linkage (Autodesk Fusion 360 design; units mm, degrees)
Autodesk Fusion 360 part; units mm, degrees
note: some values were not read from the file. Set by a fixed rule: which sketch regions a step uses.
sketch "Sketch1" plane through (0, 0, 0) normal (0, 0, 1) x (1, 0, 0)
  line L0 (15, -5) -> (-15, -5)
  line L1 (-15, -5) -> (-15, 5)
  line L2 (-15, 5) -> (15, 5)
  line L3 (15, 5) -> (15, -5)
  line L4 (15, -5) -> (-15, 5) construction
  line L5 (-15, -5) -> (15, 5) construction
  line L6 (15, 5) -> (15, 6)
  line L7 (-15, 5) -> (-15, 6)
  line L8 (-15, 6) -> (15, 6)
  circle A0 centre (15, 0) radius 5
  circle A1 centre (-15, 0) radius 5
  circle A2 centre (17.598076, -1.5) radius 0.75
  arc A3 (11.752405, -1.875) -> (18.247595, -1.875) centre (15, 0) ccw
  arc A4 (13.051443, -1.125) -> (11.752405, -1.875) centre (12.401924, -1.5) ccw
  arc A5 (13.051443, -1.125) -> (16.948557, -1.125) centre (15, 0) ccw
  arc A6 (18.247595, -1.875) -> (16.948557, -1.125) centre (17.598076, -1.5) ccw
  arc A7 (12.401924, -1.5) -> (17.598076, -1.5) centre (15, 0) ccw construction
  circle A8 centre (-15, 0) radius 1
  circle A9 centre (-13.341688, 2.5) radius 0.75
  circle A10 centre (15, 0) radius 0.85
  line L9 (10, 0) -> (10, 5)
  line L10 (10, 0) -> (10, -5)
  line L11 (-10, 0) -> (-10, 5)
  line L12 (-10, 0) -> (-10, -5)
  circle A11 centre (-13.341688, 2.5) radius 1.5
  circle A12 centre (17.598076, -1.5) radius 1.5
  spline S0 degree 5 poles (-13.906239, 3.889705) (-13.820569, 3.930394) (-13.594142, 4.00436) (-13.089374, 4.092943) (-12.082571, 4.167095) (-10.28252, 4.16815) (-7.990298, 4.046011) (-5.364162, 3.702697) (-2.588377, 3.078057) (0.216352, 2.217267) (2.95153, 1.211009) (5.549959, 0.187001) (7.964451, -0.719306) (10.166297, -1.382464) (12.141061, -1.714787) (13.885488, -1.67539) (15.098724, -1.33535) (15.908025, -0.90749) (16.403158, -0.545975) (16.639624, -0.34615) knots 0 0 0 0 0 0 0.06666667 0.13333333 0.2 0.26666667 0.33333333 0.4 0.46666667 0.53333333 0.6 0.66666667 0.73333333 0.8 0.86666667 0.93333333 1 1 1 1 1 1
  line L13 (-11.458957, 4.328773) -> (-4.541043, 3.671227)
  spline S1 degree 5 poles (-13.025243, 1.033759) (-12.77026, 1.082867) (-12.235105, 1.173979) (-11.356811, 1.289333) (-10.033525, 1.400235) (-8.132174, 1.457296) (-6.01483, 1.406336) (-3.754068, 1.195619) (-1.485479, 0.739596) (0.736265, 0.061952) (2.894168, -0.762718) (5.003407, -1.624735) (7.092733, -2.409171) (9.191281, -3.021107) (11.316096, -3.407147) (13.476739, -3.540705) (15.236985, -3.439146) (16.575337, -3.246285) (17.475584, -3.06623) (17.927711, -2.963332) knots 0 0 0 0 0 0 0.06666667 0.13333333 0.2 0.26666667 0.33333333 0.4 0.46666667 0.53333333 0.6 0.66666667 0.73333333 0.8 0.86666667 0.93333333 1 1 1 1 1 1
  line L14 (-8.520512, 1.622849) -> (-1.602599, 0.965303)
  point P0 (-8, 4)
  point P1 (9.308019, -1.092546)
  point P2 (-5.061556, 1.294076)
  point P3 (6.721235, -2.240412)
  dimension "d1" = 30
  dimension "d2" = 10
  dimension "d5" = 1
  dimension "d6" = 1
  dimension "d7" = 1.5
  dimension "d8" = 3
  dimension "d9" = 1.5
  dimension "d10" = 2
  dimension "d11" = 1.5
  dimension "d12" = 3
  dimension "d13" = 2.5
  dimension "d14" = 1.7
  dimension "d31" = 3
  dimension "d32" = 3
  constraint horizontal L0
  constraint perpendicular L0 L1
  constraint parallel L0 L2
  constraint parallel L1 L3
  constraint coincident L4 origin
  constraint coincident L5 origin
  constraint perpendicular L2 L6
  constraint perpendicular L2 L7
  constraint midpoint L3 A0.centre
  constraint coincident L0.start A0
  constraint midpoint L1 A1.centre
  constraint coincident L0.end A1
  constraint tangent A3 A4
  constraint tangent A4 A5
  constraint tangent A5 A6
  constraint tangent A3 A6
  constraint coincident A0.centre A3.centre
  constraint concentric A1 A8
  constraint concentric A0 A10
  constraint coincident A0 L9.start
  constraint coincident L2 L9.end
  constraint tangent A0 L9
  constraint perpendicular L2 L9
  constraint coincident L0 L10.end
  constraint tangent A0 L10
  constraint coincident A1 L11.start
  constraint coincident L2 L11.end
  constraint tangent A1 L11
  constraint perpendicular L2 L11
  constraint coincident L0 L12.end
  constraint tangent A1 L12
  constraint concentric A9 A11
  constraint concentric A6 A12
  constraint midpoint P0 L13
  measures "d1" distance of L1.end L2.end
  measures "d2" distance of L0.end L1.end
  measures "d5" distance of L2.end L6.end
  measures "d6" distance of L1.end L7.end
  measures "d7" diameter of A2
  measures "d10" diameter of A8
  measures "d11" diameter of A9
  measures "d14" diameter of A10
  measures "d31" diameter of A11
  measures "d32" diameter of A12
extrude "Extrude7" add sketch "Sketch1" along normal blind 4 contours A2 A3 A5 A6 A12 | A0 L10 S0 S1 | A0 A3 A4 S0 S1 | L10 L11 S0 S1 | L3 A3 A4 A5 S0 S1 | L3 A3 A5 A12 S1 | A3 A12 S1 | L3 A5 S0 | L3 A5 A12 S0 | A2 A3 A5 A12 | A1 A11 S0 S1 | A1 L11 S0 S1 | A11 picked at (18.306984, -2.225643) picked at (10.508254, -2.804031) picked at (10.881569, -1.979998) picked at (-7.687185, 2.224083) picked at (14.341357, -3.022923) picked at (15.681946, -2.680596) picked at (17.334812, -2.998384) picked at (14.863156, -1.654736) picked at (15.395632, -1.500858) picked at (17.37711, -2.592378) picked at (-11.025428, 2.2525) picked at (-10.637546, 3.32386) picked at (-13.909485, 3.610058)
extrude "Extrude8" cut 1 faces at (-7.687185, 2.224083, 4) along direction (0, 0, -1) blind 0.3
extrude "Extrude9" [suppressed]
extrude "Extrude1" [suppressed]
ref_plane "WorkPlane1" through (2.5, 0.5, 5) normal (0, 0, 1) x (1, 0, 0)
extrude "Extrude2" [suppressed]
extrude "Extrude3" [suppressed]
fillet "Fillet1" [suppressed]
extrude "Extrude4" [suppressed]
extrude "Extrude5" [suppressed]
extrude "Extrude6" [suppressed]
equation "d1 = length"
equation "d2 = thickness"
equation "length = 30 mm"
equation "thickness = 10 mm"
equation "d7 = 1.8 mm - gap"
equation "d11 = 1.8 mm - gap"
equation "d14 = 2 mm - gap"
equation "gap = 0.3 mm"
